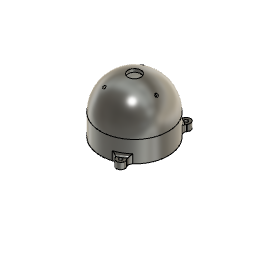
SensorHolder_top_V1_0 (Autodesk Fusion 360 design; units mm, degrees)
Autodesk Fusion 360 part; units mm, degrees
sketch "Sketch1" plane through (0, 0, 15) normal (0, 0, 1) x (-1, 0, 0)
  arc A0 (-14.673939, 33.097217) -> (-21.602142, 29.097217) centre (-18.13804, 31.097217) ccw
  line L0 (-21.602142, 29.097217) -> (-21.133716, 28.285878)
  arc A1 (-21.864726, 23.365225) -> (-21.133716, 28.285878) centre (-24.597817, 26.285878) ccw
  arc A2 (-21.864726, 23.365225) -> (-21.651614, -23.562844) centre (0, 0) ccw
  arc A3 (-20.893965, -28.508199) -> (-21.651614, -23.562844) centre (-24.358066, -26.508199) ccw
  line L1 (-20.893965, -28.508199) -> (-21.326061, -29.256612)
  arc A4 (-21.326061, -29.256612) -> (-14.397858, -33.256612) centre (-17.86196, -31.256612) ccw
  line L2 (-14.397858, -33.256612) -> (-13.929431, -32.445274)
  arc A5 (-9.302515, -30.618021) -> (-13.929431, -32.445274) centre (-10.46533, -34.445274) ccw
  arc A6 (-9.302515, -30.618021) -> (31.231828, -6.969426) centre (0, 0) ccw
  arc A7 (35.135807, -3.840605) -> (31.231828, -6.969426) centre (35.135807, -7.840605) ccw
  line L3 (35.135807, -3.840605) -> (36, -3.840605)
  arc A8 (36, -3.840605) -> (36, 4.159395) centre (36, 0.159395) ccw
  line L4 (36, 4.159395) -> (35.063147, 4.159395)
  arc A9 (31.167242, 7.252796) -> (35.063147, 4.159395) centre (35.063147, 8.159395) ccw
  arc A10 (31.167242, 7.252796) -> (-9.580214, 30.53227) centre (0, 0) ccw
  arc A11 (-14.241842, 32.348804) -> (-9.580214, 30.53227) centre (-10.777741, 34.348804) ccw
  line L5 (-14.241842, 32.348804) -> (-14.673939, 33.097217)
  circle A12 centre (-17.86196, -31.256612) radius 1.6
  circle A13 centre (-18.138041, 31.097217) radius 1.6
  circle A14 centre (36, 0.159395) radius 1.6
  circle A15 centre (12.84, 0) radius 8.14
  circle A16 centre (-12.66, 0) radius 8.14
  arc A17 (-9.302515, -30.618021) -> (31.231828, -6.969426) centre (0, 0) ccw
  arc A18 (35.135807, -3.840605) -> (31.231828, -6.969426) centre (35.135807, -7.840605) ccw
  arc A19 (36, -3.840605) -> (36, 4.159395) centre (36, 0.159395) ccw
  arc A20 (31.167242, 7.252796) -> (35.063147, 4.159395) centre (35.063147, 8.159395) ccw
  line L6 (36, 4.159395) -> (35.063147, 4.159395)
  line L7 (36, -3.840605) -> (35.135807, -3.840605)
  arc A21 (31.167242, 7.252796) -> (-9.580214, 30.53227) centre (0, 0) ccw
  arc A22 (-14.241842, 32.348804) -> (-9.580214, 30.53227) centre (-10.777741, 34.348804) ccw
  line L8 (-14.673939, 33.097217) -> (-14.241842, 32.348804)
  arc A23 (-14.673939, 33.097217) -> (-21.602142, 29.097217) centre (-18.13804, 31.097217) ccw
  line L9 (-21.602142, 29.097217) -> (-21.133716, 28.285878)
  arc A24 (-21.864726, 23.365225) -> (-21.133716, 28.285878) centre (-24.597817, 26.285878) ccw
  circle A25 centre (-18.138041, 31.097217) radius 1.6
  circle A26 centre (36, 0.159395) radius 1.6
  arc A27 (-9.302515, -30.618021) -> (-13.929431, -32.445274) centre (-10.46533, -34.445274) ccw
  line L10 (-14.397858, -33.256612) -> (-13.929431, -32.445274)
  arc A28 (-21.326061, -29.256612) -> (-14.397858, -33.256612) centre (-17.86196, -31.256612) ccw
  arc A29 (-20.893965, -28.508199) -> (-21.651614, -23.562844) centre (-24.358066, -26.508199) ccw
  line L11 (-21.326061, -29.256612) -> (-20.893965, -28.508199)
  arc A30 (-21.864726, 23.365225) -> (-21.651614, -23.562844) centre (0, 0) ccw
  circle A31 centre (-17.86196, -31.256612) radius 1.6
  circle A32 centre (0, 0) radius 29
extrude "Extrude1" add sketch "Sketch1" along normal blind 6 contours A0 L0 A1 A2 A3 L1 A4 L2 A5 A6 A7 L3 A8 L4 A9 A10 A11 L5 A17 A18 A19 A20 L6 L7 A21 A22 L8 A23 L9 A24 A27 L10 A28 A29 L11 A30 picked at (-17.533676, -27.072144)
sketch "Sketch2" plane through (0, 0, 21) normal (0, 0, 1) x (-1, 0, 0)
  circle A0 centre (-17.86196, -31.256612) radius 1.6
  circle A1 centre (0, 0) radius 29
  circle A2 centre (-18.138041, 31.097217) radius 1.6
  circle A3 centre (36, 0.159395) radius 1.6
  arc A4 (-14.673939, 33.097217) -> (-21.602142, 29.097217) centre (-18.13804, 31.097217) ccw
  line L0 (-21.602142, 29.097217) -> (-21.133716, 28.285878)
  arc A5 (-21.864726, 23.365225) -> (-21.133716, 28.285878) centre (-24.597817, 26.285878) ccw
  arc A6 (-21.864726, 23.365225) -> (-21.651614, -23.562844) centre (0, 0) ccw
  arc A7 (-20.893965, -28.508199) -> (-21.651614, -23.562844) centre (-24.358066, -26.508199) ccw
  line L1 (-20.893965, -28.508199) -> (-21.326061, -29.256612)
  arc A8 (-21.326061, -29.256612) -> (-14.397858, -33.256612) centre (-17.86196, -31.256612) ccw
  line L2 (-14.397858, -33.256612) -> (-13.929431, -32.445274)
  arc A9 (-9.302515, -30.618021) -> (-13.929431, -32.445274) centre (-10.46533, -34.445274) ccw
  arc A10 (-9.302515, -30.618021) -> (31.231828, -6.969426) centre (0, 0) ccw
  arc A11 (35.135807, -3.840605) -> (31.231828, -6.969426) centre (35.135807, -7.840605) ccw
  line L3 (35.135807, -3.840605) -> (36, -3.840605)
  arc A12 (36, -3.840605) -> (36, 4.159395) centre (36, 0.159395) ccw
  line L4 (36, 4.159395) -> (35.063147, 4.159395)
  arc A13 (31.167242, 7.252796) -> (35.063147, 4.159395) centre (35.063147, 8.159395) ccw
  arc A14 (31.167242, 7.252796) -> (-9.580214, 30.53227) centre (0, 0) ccw
  arc A15 (-14.241842, 32.348804) -> (-9.580214, 30.53227) centre (-10.777741, 34.348804) ccw
  line L5 (-14.241842, 32.348804) -> (-14.673939, 33.097217)
  circle A16 centre (0, 0) radius 29
  circle A17 centre (0, 0) radius 32
extrude "Extrude2" add sketch "Sketch2" along normal blind 14 contours A6 A10 A14 A17 picked at (29.538785, 9.206455)
fillet "Fillet1" radius 2.25 3 edges at (16.125684, -27.639868, 21) (-31.99967, -0.145318, 21) (15.873986, 27.785186, 21)
sketch "Sketch3" plane through (0, 0, 0) normal (1, 0, 0) x (0, 1, 0)
  line L0 (32, 35) -> (-32, 35) construction
  line L1 (0, 81.000001) -> (0, 57.000001) construction
  circle A0 centre (0, 35) radius 32
  line L2 (0, 35) -> (32, 35)
  line L3 (0, 35) -> (0, 67)
  circle A1 centre (0, 35) radius 29
  dimension "d96" = 3
  constraint perpendicular L0 L1
  constraint midpoint L0 A0.centre
  constraint coincident L0.start A0
  constraint coincident A0.centre L2.start
  constraint coincident L0.start L2.end
  constraint coincident A0 L3.end
  constraint perpendicular L0 L3
  constraint concentric A0 A1
  measures "d96" distance of A0 A1
revolve "Revolve1" add sketch "Sketch3" angle 360 about axis through (0, 0, 15) along (0, 0, -1) contours A0 L2 L3 A1 picked at (1.518025, 65.891429)
ref_plane "WorkPlane1" through (0, 0, 67) normal (0, 0, 1) x (1, 0, 0)
sketch "Sketch4" plane through (0, 0, 67) normal (0, 0, 1) x (1, 0, 0)
  circle A0 centre (0, 0) radius 6
  dimension "d99" = 12
  constraint coincident A0.centre origin
  measures "d99" diameter of A0
extrude "Extrude3" cut sketch "Sketch4" along normal up to surface contours A0 picked at (0.405498, -1.776603) end surface at (-21.345827, -19.262073, 38.78526)
sketch "Sketch5" plane through (0, 0, 0) normal (0, 1, 0) x (1, 0, 0)
  line L0 (0.339643, -38.660358) -> (28.339643, -66.660358) construction
  line L1 (0, -67) -> (0, -3) construction
  line L2 (22.856942, -61.177657) -> (23.846892, -60.187708)
  line L3 (23.846892, -60.187708) -> (20.311358, -56.652174)
  line L4 (20.311358, -56.652174) -> (18.331459, -58.632073)
  line L5 (18.331459, -58.632073) -> (21.866993, -62.167607)
  line L6 (21.866993, -62.167607) -> (22.856942, -61.177657)
  line L7 (22.856942, -61.177657) -> (19.321408, -57.642123)
  point P0 (22.856942, -61.177657)
  dimension "d102" = 45
  dimension "d103" = 5
  dimension "d107" = 2.8
  constraint perpendicular L0 L2
  constraint perpendicular L2 L3
  constraint perpendicular L0 L4
  constraint perpendicular L2 L5
  constraint perpendicular L0 L6
  constraint symmetric L0 L3 L5
  measures "d102" angle of L0 L1
revolve "Revolve2" cut sketch "Sketch5" angle 360 about axis through (0.339643, 0, 38.660358) along (0.70710678, 0, 0.70710678) contours L4 L5 L6 L7 picked at (19.839953, -59.480601)
pattern_circular "C-Pattern1" count 3 over 360 about axis through (0, 0, 15) along (0, 0, 1) of "Revolve2"
